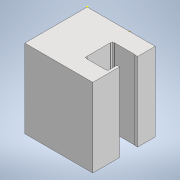
# Autodesk Inventor part: Z Belt 2
Saved by Autodesk Inventor 2022 (Build 260153000, 153)
## iProperties
Created: 2022-02-24
Part Number: Z Belt 2
Material: Generic
Document SubType Name: Modeling
Designer: Nicoli
Density: 1 g/cm^3
Appearance: Default
Author: Nicoli
Autodesk Inventor part; units mm, degrees
ref_plane "YZ Plane" through (0, 0, 0) normal (1, 0, 0) x (0, 1, 0)
ref_plane "XZ Plane" through (0, 0, 0) normal (0, 1, 0) x (-1, 0, 0)
ref_plane "XY Plane" through (0, 0, 0) normal (0, 0, 1) x (1, 0, 0)
sketch "Sketch1" plane through (0, 0, 0) normal (0, 0, 1) x (1, 0, 0)
  line L0 (-24.03, -44) -> (-24.03, 0)
  line L1 (-46, 9.9228) -> (-46, 9.9228)
  line L2 (-24.03, 0) -> (-24.03, -38.7439)
  line L3 (-24.03, -38.7439) -> (-24.03, -44)
  line L4 (-24.03, -44) -> (0, -44)
  line L5 (0, -44) -> (0, 0)
  line L6 (0, 0) -> (-24.03, 0)
  line L7 (-24.03, 0) -> (-24.03, -5.2561)
  line L8 (-24.03, -5.2561) -> (-24.03, -44)
  dimension "d3" = 44
  dimension "d57" = 24.03
  constraints: 18 end point, 4 vertical, 2 equal length, 1 coincident, 1 collinear, 1 horizontal, 1 perpendicular
  measures "d3" distance of L4.end L5.end
  measures "d57" distance between parallel lines of L5 L8
extrude "Extrusion1" add sketch "Sketch1" along normal blind 35
sketch "Sketch2" plane through (0, -44, 0) normal (1, 0, 0) x (0, 0, -1)
  line L0 (0.4959, 44) -> (-35, 44)
  line L1 (-35, 44) -> (-25, 44)
  line L2 (-25, 44) -> (-25, 0)
  line L3 (-25, 0) -> (-35, 0)
  line L4 (-35, 0) -> (-35, 44)
  line L5 (0, 0) -> (-10, 0)
  line L6 (-10, 0) -> (-10, 44)
  line L7 (-10, 44) -> (0, 44)
  line L8 (0, 44) -> (0, 0)
  line L9 (0, 44) -> (-35, 44) projected
  line L10 (0, 0) -> (-35, 0) projected
  point P0 (-14, 8.5)
  point P1 (-10, 44)
  point P2 (-14, 8.5)
  dimension "d6" = 10
  dimension "d7" = 10
  dimension "d30" = 4
  dimension "d59" = 8.5
  constraints: 18 end point, 4 parallel, 2 horizontal, 2 perpendicular, 1 coincident, 1 collinear, 1 point on line
  measures "d6" distance of L2.end L3.end
  measures "d7" distance of L6.end L7.end
  measures "d30" distance from line of L6 point (-14, 8.5)
  measures "d59" distance from line of L10 point (-14, 8.5)
extrude "Extrusion2" add sketch "Sketch2" along normal blind 16.6 contours L8 L5 L6 L0 | L2 L3 L4 L0
hole "Hole2" at (0, -35.5, 14) direction (-1, 0, 0) diameter 4 depth 6
ref_plane "Work Plane1" through (-40, -10, 25) normal (0, 1, 0) x (1, 0, 0)
sketch "Sketch6" plane through (0, -44, 25) normal (0, 0, -1) x (-1, 0, 0)
  line L0 (0, 44) -> (0, 0) projected
  line L1 (0, 44) -> (-16.6, 44) projected
  line L2 (-16.6, 0) -> (-16.6, 44) projected
  line L3 (0, 0) -> (-16.6, 0) projected
  line L4 (-16.6, 44) -> (-16.6, 0) projected
  line L5 (0, 0) -> (-16.6, 0) projected
  line L6 (-16.6, 44) -> (-12.6, 44)
  line L7 (-12.6, 44) -> (-12.6, 0)
  line L8 (-12.6, 0) -> (-16.6, 0)
  line L9 (-16.6, 0) -> (-16.6, 44)
  dimension "d40" = 4
  constraints: 8 end point, 2 parallel, 1 horizontal, 1 perpendicular, 1 point on line
  measures "d40" distance of L7.end L8.end
extrude "Extrusion6" add sketch "Sketch6" along normal blind 5 contours L7 L3 L2 L1
thicken "Thicken1" operation add thickness 0.1 both sides no extend neighbours yes toward (0, 0, 1) faces at (8.4, -14.6667, 25) (5.5333, -14.6667, 10)
sketch "Sketch7" plane through (21.97, 0, 35) normal (0, 1, 0) x (1, 0, 0)
  line L0 (-21.97, 25.1) -> (-21.97, 9.9) projected
  line L1 (-22.17, 10.9) -> (-21.97, 10.9)
  line L2 (-21.97, 10.9) -> (-21.97, 24.1)
  line L3 (-21.97, 24.1) -> (-22.17, 24.1)
  line L4 (-22.17, 24.1) -> (-22.17, 10.9)
  line L5 (-21.97, 25.1) -> (-5.37, 25.1) projected
  line L6 (-20.97, 25.1) -> (-9.37, 25.1)
  line L7 (-9.37, 25.1) -> (-9.37, 25.3)
  line L8 (-9.37, 25.3) -> (-20.97, 25.3)
  line L9 (-20.97, 25.3) -> (-20.97, 25.1)
  line L10 (-21.97, 9.9) -> (-9.37, 9.9) projected
  line L11 (-20.97, 9.9) -> (-10.37, 9.9)
  line L12 (-10.37, 9.9) -> (-10.37, 9.7)
  line L13 (-10.37, 9.7) -> (-20.97, 9.7)
  line L14 (-20.97, 9.7) -> (-20.97, 9.9)
  line L15 (-9.37, 9.9) -> (-9.37, 15) projected
  point P0 (-21.97, 35)
  dimension "d45" = 1
  dimension "d46" = 1
  dimension "d47" = 0.2
  dimension "d48" = 0.2
  dimension "d49" = 1
  dimension "d50" = 1
  dimension "d51" = 0.2
  constraints: 24 end point, 6 parallel, 4 point on line, 3 horizontal, 3 perpendicular, 1 collinear
  measures "d45" distance between parallel lines of L15 L12
  measures "d46" distance between parallel lines of L0 L14
  measures "d47" distance of L13.end L11.start
  measures "d48" distance between parallel lines of L2 L4
  measures "d49" distance between parallel lines of L1 L10
  measures "d50" distance between parallel lines of L3 L5
  measures "d51" distance of L8.end L6.start
extrude "Extrusion7" cut sketch "Sketch7" against normal through all
sketch "Sketch8" plane through (21.97, 0, 35) normal (0, 1, 0) x (1, 0, 0)
  line L0 (-7.87, -2.812) -> (-1.3086, -2.812)
  line L1 (-1.3086, -2.812) -> (-1.3086, 42.7261)
  line L2 (-1.3086, 42.7261) -> (-7.87, 42.7261)
  line L3 (-7.87, 42.7261) -> (-7.87, -2.812)
  line L4 (-9.37, 9.9) -> (-9.37, 15) projected
  point P0 (-21.97, 35)
  dimension "d54" = 1.5
  constraints: 8 end point, 2 parallel, 1 horizontal, 1 perpendicular
  measures "d54" distance between parallel lines of L3 L4
extrude "Extrusion8" cut sketch "Sketch8" against normal through all
sketch "Sketch9" plane through (-24.03, -44, 0) normal (-1, 0, 0) x (0, 0, 1)
  circle A0 centre (19.382, 22) radius 1.7
  circle A1 centre (9.382, 22) radius 1.7
  line L0 (0, 44) -> (0, 0) projected
  line L1 (0, 0) -> (35, 0) projected
  dimension "d60" = 10
  dimension "d61" = 9.382
  dimension "d62" = 22
  constraints: 2 centre point, 1 horizontal alignment
  measures "d60" distance of A0.centre A1.centre
  measures "d61" distance from line of L0 A1.centre
  measures "d62" distance from line of L1 A1.centre
hole "Hole3" at (-24.03, -22, 9.382) at (-24.03, -22, 19.382) direction (1, 0, 0) diameter 4 depth 10
body "Solid1"
